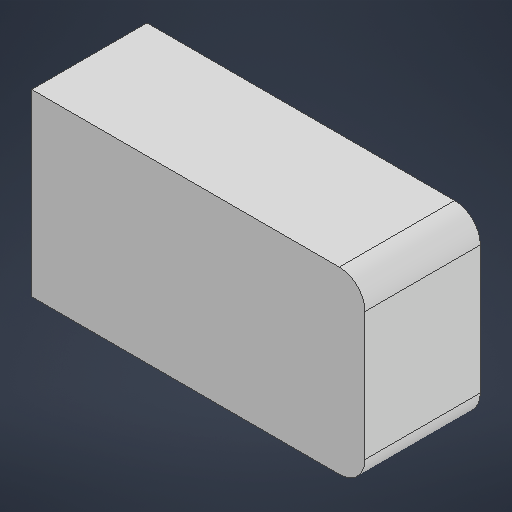
# Autodesk Inventor part: P_Case
Saved by Autodesk Inventor 2026 (Build 300175000, 175)
## iProperties
Created: 2025-09-05
Part Number: P_Case
Material: Generisch
Document SubType Name: Modeling
Designer: FAL
Density: 1 g/cm^3
Appearance: Vorgabe
Mass: 1.16843 g
Surface Area: 17.0683 cm^2
Volume: 1.16843 cm^3
Author: FAL
Autodesk Inventor part; units mm, degrees
ref_plane "YZ Plane" through (0, 0, 0) normal (1, 0, 0) x (0, 1, 0)
ref_plane "XZ Plane" through (0, 0, 0) normal (0, 1, 0) x (-1, 0, 0)
ref_plane "XY Plane" through (0, 0, 0) normal (0, 0, 1) x (1, 0, 0)
sketch "Skizze1" plane through (0, 0, 0) normal (0, 1, 0) x (-1, 0, 0)
  line L0 (13, 7) -> (-13, 7)
  line L1 (-13, 7) -> (-13, -7)
  line L2 (-13, -7) -> (13, -7)
  line L3 (13, -7) -> (13, 7)
  line L4 (13, 7) -> (-13, -7) construction
  line L5 (-13, 7) -> (13, -7) construction
  point P0 (0, 0)
  dimension "d0" = 14
  dimension "d2" = 26
  constraints: 12 end point, 2 midpoint, 2 parallel, 1 horizontal, 1 perpendicular
  measures "d0" distance between parallel lines of L2 L0
  measures "d2" distance between parallel lines of L3 L1
extrude "Extrusion1" add sketch "Skizze1" along normal blind 9
fillet "Rundung1" radius 2 2 edges at (13, 4.5, 7) (13, 4.5, -7)
shell "Wandung1" thickness 1.5 removed faces 2 at (3, 9, 2.3333) at (-13, 6, -2.3333)
sketch "Skizze5" plane through (0, 9, 0) normal (0, 1, 0) x (1, 0, 0)
  line L0 (10.5, 5.5) -> (11.5, 5.5)
  line L1 (11.5, 5.5) -> (11.5, -5.5)
  line L2 (11.5, -5.5) -> (10.5, -5.5)
  line L3 (10.5, -5.5) -> (10.5, 5.5)
  line L4 (11.5, 5) -> (11.5, -5) projected
  line L5 (-13, 5.5) -> (11, 5.5) projected
  line L6 (11, -5.5) -> (-13, -5.5) projected
  point P0 (0, 0)
  dimension "d15" = 1
  constraints: 8 end point, 3 collinear, 2 parallel, 1 horizontal, 1 perpendicular
  measures "d15" distance between parallel lines of L1 L3
extrude "Extrusion3" add sketch "Skizze5" against normal blind 2
